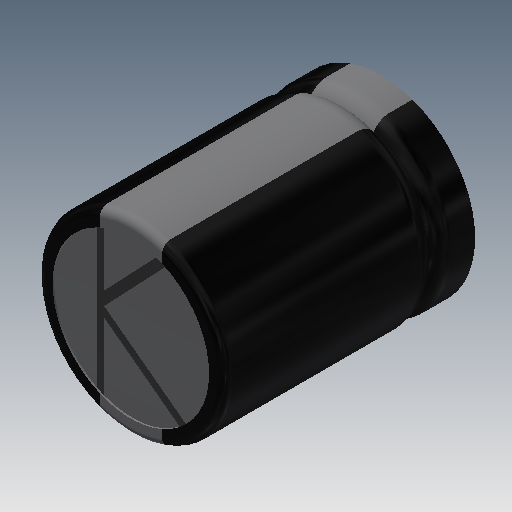
# Autodesk Inventor part: config - capasitor 3500 μF
Saved by Autodesk Inventor 2020 (Build 240152000, 152)
## iProperties
Created: 2005-12-06
Part Number: config - capasitor 3500 μF
Document SubType Name: Modeling
Designer: Simon.Ng@autodesk.com
Stock Number: config - capasitor 3500 μF
Density: 1 g/cm^3
Material: Generic
Mass: 1.78807 g
Surface Area: 8.36933 cm^2
Volume: 1.78807 cm^3
Appearance: Glossy - Black
Company: Autodesk Asia Pte. Ltd.
Title: PC Demo
Author: Simon.Ng@autodesk.com
Autodesk Inventor part; units mm, degrees
ref_plane "YZ Plane" through (0, 0, 0) normal (1, 0, 0) x (0, 1, 0)
ref_plane "XZ Plane" through (0, 0, 0) normal (0, 1, 0) x (-1, 0, 0)
sketch "Sketch1" plane through (0, 0, 0) normal (0, 0, 1) x (1, 0, 0)
  line L0 (0, 9.6) -> (0, -7.2) construction
  line L1 (-7.2, 0) -> (9.6, 0) construction
  circle A0 centre (0, 0) radius 6
  dimension "d0" = 12
  constraints: 2 point on line, 1 centre point
  measures "d0" diameter of A0
extrude "Extrusion1" add sketch "Sketch1" along normal blind 16
sketch "Sketch6" plane through (0, 0, 0) normal (1, 0, 0) x (0, 1, 0)
  line L0 (0, 20.8) -> (0, -1.6) projected
  line L1 (6, 0) -> (6, 16) projected
  line L2 (6, 3.5) -> (6, 1.5)
  line L3 (6, 2.5) -> (5.5, 2.5) construction
  line L4 (-6, 0) -> (6, 0) construction
  arc A0 (5.5, 2.5) -> (6, 3.5) centre (4.75, 3.5) ccw
  arc A1 (6, 1.5) -> (5.5, 2.5) centre (4.75, 1.5) ccw
  point P0 (0, 0)
  dimension "d16" = 2
  dimension "d17" = 2.5
  dimension "d18" = 0.5
  constraints: 4 end point, 4 point on circle, 2 centre point, 2 point on line, 2 tangent, 1 collinear, 1 horizontal, 1 midpoint
  measures "d16" distance of L2.start L2.end
  measures "d17" distance between parallel lines of L4 L3
  measures "d18" distance of L3.start L3.end
revolve "Revolution1" cut sketch "Sketch6" angle 360 about axis through (0, 0, 0) along (0, 0, -1)
sketch "Sketch2" plane through (0, 0, 16) normal (0, 0, 1) x (1, 0, 0)
  circle A0 centre (0, 0) radius 6 projected
  circle A1 centre (0, 0) radius 5
  dimension "d3" = 1
  constraints: 1 centre point, 1 coincident
  measures "d3" radial gap between concentric circles of A1 A0
extrude "Extrusion2" cut sketch "Sketch2" against normal blind 0.1 contours A1
sketch "Sketch3" plane through (0, 0, 15.9) normal (0, 0, 1) x (1, 0, 0)
  line L0 (-2.2779, 4.6629) -> (-1.8048, 4.6629)
  line L1 (-1.8048, 4.6629) -> (-1.8048, -4.9424)
  line L2 (-1.8048, -4.9424) -> (-2.2779, -4.9424)
  line L3 (-2.2779, -4.9424) -> (-2.2779, 4.6629)
  line L4 (-1.8048, 0.2777) -> (-2.233, 0.6841)
  line L5 (-2.233, 0.6841) -> (1.932, 5.0712)
  line L6 (1.932, 5.0712) -> (2.3602, 4.6648)
  line L7 (2.3602, 4.6648) -> (-1.8048, 0.2777)
  line L8 (-1.8048, 0.2777) -> (-2.1189, -0.1414)
  line L9 (-2.1189, -0.1414) -> (3.111, -4.0616)
  line L10 (3.111, -4.0616) -> (3.4251, -3.6426)
  line L11 (3.4251, -3.6426) -> (-1.8048, 0.2777)
  circle A0 centre (0, 0) radius 5 projected
  constraints: 24 end point, 6 parallel, 3 perpendicular, 2 point on circle, 1 horizontal, 1 point on line
extrude "Extrusion3" cut sketch "Sketch3" against normal blind 0.05 contours L0 A0 L3 | L1 L5 L4 L8 L9 A0 L3 | L5 A0 L7 L1 | L1 L4 L5 | L5 L6 L7 A0 | A0 L1 L2 L3 | L11 A0 L9 L1 | L1 L9 L8 | L10 L9 A0
fillet "Fillet1" radius 0.5 1 edges at (-6, 0, 16)
sketch "Sketch5" plane through (0, 0, 16) normal (0, 0, 1) x (1, 0, 0)
  circle A0 centre (0, 0) radius 5 projected
  circle A1 centre (0, 0) radius 6 projected
  line L0 (2, -4.5826) -> (2, -7)
  line L1 (2, -7) -> (-2, -7)
  line L2 (-2, -7) -> (-2, -4.5826)
  line L3 (0, -7.2) -> (0, 9.6) projected
  point P0 (0, -6)
  point P1 (0, -6)
  dimension "d12" = 1
  dimension "d13" = 4
  constraints: 6 end point, 2 point on circle, 1 coincident, 1 parallel, 1 point on line, 1 vertical alignment, 2 other
  measures "d12" distance from line of L1 point (0, -6)
  measures "d13" distance of L0.end L1.end
split_face "Split1"
ref_plane "Work Plane1" through (10, 0, 0) normal (1, 0, 0) x (0, 1, 0)
body "Solid1"
